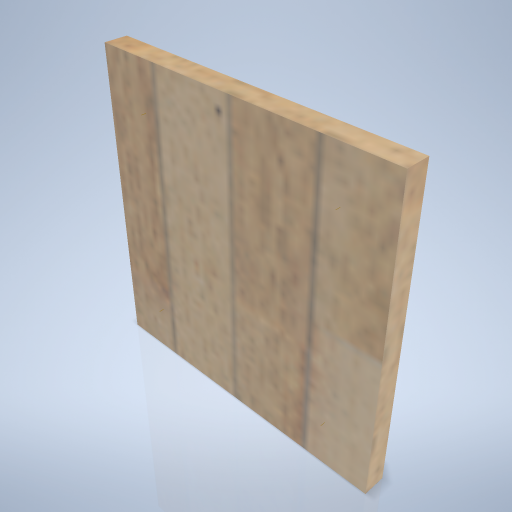
# Autodesk Inventor part: wooden support
Saved by Autodesk Inventor 2024.2 (Build 282272000, 272)
## iProperties
Created: 2024-05-14
Part Number: wooden support
Material: Holz (Ahorn)
Document SubType Name: Modeling
Designer: Fabri
Density: 0.67 g/cm^3
Appearance: Ahorn - natur - glänzend - dunkel getönt
Author: Fabri
Autodesk Inventor part; units mm, degrees
ref_plane "YZ Plane" through (0, 0, 0) normal (1, 0, 0) x (0, 1, 0)
ref_plane "XZ Plane" through (0, 0, 0) normal (0, 1, 0) x (-1, 0, 0)
ref_plane "XY Plane" through (0, 0, 0) normal (0, 0, 1) x (1, 0, 0)
sketch "Skizze1" plane through (0, 0, 0) normal (0, 1, 0) x (-1, 0, 0)
  line L0 (-100, 100) -> (100, 100)
  line L1 (100, 100) -> (100, -100)
  line L2 (100, -100) -> (-100, -100)
  line L3 (-100, -100) -> (-100, 100)
  line L4 (-100, 100) -> (100, -100) construction
  line L5 (100, 100) -> (-100, -100) construction
  point P0 (0, 0)
  dimension "d0" = 200
  dimension "d1" = 200
  constraints: 12 end point, 2 midpoint, 2 parallel, 1 horizontal, 1 perpendicular
  measures "d0" distance of L0.end L1.end
  measures "d1" distance of L1.end L2.end
extrude "Extrusion1" add sketch "Skizze1" along normal blind 25
chamfer "Fasen1" distance 10 angle 45 4 edges at (100, 25, 0) (0, 25, 100) (0, 25, -100) (-100, 25, 0)
sketch "Skizze2" plane through (0, 25, 0) normal (0, 1, 0) x (1, 0, 0)
  point P0 (0, 0)
  point P1 (0, 0)
  constraints: 2 coincident
hole "Bohrung1" at (0, 25, 0) direction (0, -1, 0) diameter 53 depth 3
sketch "Skizze3" plane through (0, 25, 0) normal (0, 1, 0) x (1, 0, 0)
  line L0 (90, -90) -> (-90, -90) projected
  line L1 (0, -90) -> (0, 90) construction
  line L2 (-90, 90) -> (90, 90) projected
  line L3 (-90, -90) -> (-90, 90) projected
  line L4 (-90, 0) -> (90.2684, 0) construction
  point P0 (0, 0)
  point P1 (-68.5, -68.5)
  point P2 (68.5, -68.5)
  point P3 (68.5, 68.5)
  point P4 (-68.5, 68.5)
  point P5 (0.1342, 0)
  dimension "d21" = 68.5
  dimension "d22" = 68.5
  dimension "d23" = 137
  dimension "d24" = 68.5
  dimension "d25" = 68.5
  constraints: 4 end point, 4 midpoint, 2 horizontal alignment, 2 vertical alignment, 1 horizontal, 1 symmetric about line
  measures "d21" horizontal distance of point (0, 0) point (68.5, -68.5)
  measures "d22" horizontal distance of point (0, 0) point (-68.5, -68.5)
  measures "d23" distance of point (-68.5, 68.5) point (-68.5, -68.5)
  measures "d24" distance from line of L4 point (-68.5, -68.5)
  measures "d25" vertical distance of point (-68.5, 68.5) point (0.134, 0)
hole "Bohrung2" at (-68.5, 25, 68.5) at (68.5, 25, 68.5) at (68.5, 25, -68.5) at (-68.5, 25, -68.5) direction (0, -1, 0) diameter 8 depth 3
